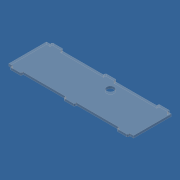
# Autodesk Inventor part: P1704_203
Saved by Autodesk Inventor 2015 (Build 190159000, 159)
## iProperties
Created: 2017-02-08
Part Number: P1704_203
Project: Manette
Material: Plastique PMMA
Description: Paroi avant - Table
Document SubType Name: Modeling
Designer: Alexandre.PICOTTE
Authority: 172x58x3
Density: 1.188 g/cm^3
Appearance: Transparent - Clair
Mass: 33.2535 g
Surface Area: 202.588 cm^2
Volume: 27.9912 cm^3
Material number: ---
Author: Boris.GAUDARD
Autodesk Inventor part; units mm, degrees
ref_plane "Plan YZ" through (0, 0, 0) normal (1, 0, 0) x (0, 1, 0)
ref_plane "Plan XZ" through (0, 0, 0) normal (0, 1, 0) x (-1, 0, 0)
ref_plane "Plan XY" through (0, 0, 0) normal (0, 0, 1) x (1, 0, 0)
sketch "Esquisse12" plane through (0, 0, 0) normal (0, 0, 1) x (1, 0, 0)
  line L0 (-86, -26) -> (-86, 26)
  line L1 (-86, 26) -> (-81, 26)
  line L2 (-81, 26) -> (-81, 29)
  line L3 (-81, 29) -> (-66, 29)
  line L4 (-66, 29) -> (-66, 26)
  line L5 (7.5, 26) -> (7.5, 29)
  line L6 (7.5, 29) -> (-7.5, 29)
  line L7 (-7.5, 29) -> (-7.5, 26)
  line L8 (66, 26) -> (66, 29)
  line L9 (66, 29) -> (81, 29)
  line L10 (81, 29) -> (81, 26)
  line L11 (81, 26) -> (86, 26)
  line L12 (86, 26) -> (86, -26)
  line L13 (86, -26) -> (81, -26)
  line L14 (81, -26) -> (81, -29)
  line L15 (81, -29) -> (66, -29)
  line L16 (66, -29) -> (66, -26)
  line L17 (-7.5, -26) -> (-7.5, -29)
  line L18 (7.5, -29) -> (7.5, -26)
  line L19 (-66, -26) -> (-66, -29)
  line L20 (-81, -29) -> (-81, -26)
  line L21 (-86, -26) -> (-81, -26)
  line L22 (-81, -29) -> (-66, -29)
  line L23 (7.5, -29) -> (-7.5, -29)
  line L24 (-66, 26) -> (-7.5, 26)
  line L25 (7.5, 26) -> (66, 26)
  line L26 (7.5, -26) -> (66, -26)
  line L27 (-7.5, -26) -> (-66, -26)
  line L28 (-120.4, 0) -> (120.4, 0) construction
  line L29 (0, -40.6) -> (0, 40.6) construction
  point P0 (0, 0)
  dimension "d86" = 52
  dimension "d87" = 3
  dimension "d88" = 5
  dimension "d90" = 15
  dimension "d112" = 172
  constraints: 56 end point, 27 point on line, 10 perpendicular, 7 equal length, 3 collinear, 2 parallel, 2 vertical, 1 horizontal, 2 other
  measures "d86" distance of L0.start L0.end
  measures "d87" distance of L1.end L2.end
  measures "d88" distance of L0.end L1.end
  measures "d90" distance of L2.end L3.end
  measures "d112" distance between parallel lines of L12 L0
extrude "Extrusion5" add sketch "Esquisse12" along normal blind 3
sketch "Esquisse13" plane through (0, 0, 3) normal (0, 0, 1) x (1, 0, 0)
  point P0 (0, 0)
  point P1 (-81, 26)
  point P2 (-66, 26)
  point P3 (-81, -26)
  point P4 (-66, -26)
  point P5 (-7.5, -26)
  point P6 (7.5, -26)
  point P7 (66, -26)
  point P8 (81, -26)
  point P9 (81, 26)
  point P10 (66, 26)
  point P11 (-7.5, 26)
  point P12 (7.5, 26)
hole "Perçage6" at (-81, 26, 3) at (-66, 26, 3) at (-81, -26, 3) at (-66, -26, 3) at (-7.5, -26, 3) at (7.5, -26, 3) at (66, -26, 3) at (81, -26, 3) at (81, 26, 3) at (66, 26, 3) at (-7.5, 26, 3) at (7.5, 26, 3) direction (0, 0, -1) diameter 1 end through all
chamfer "Chanfrein3" distance 1 angle 45 12 edges at (-81, 29, 1.5) (-66, 29, 1.5) (-7.5, 29, 1.5) (7.5, 29, 1.5) (66, 29, 1.5) (81, 29, 1.5) (-81, -29, 1.5) (-66, -29, 1.5) (-7.5, -29, 1.5) (7.5, -29, 1.5) (66, -29, 1.5) (81, -29, 1.5)
sketch "Esquisse14" plane through (0, 0, 3) normal (0, 0, 1) x (1, 0, 0)
  circle A0 centre (14.3, 13.8) radius 5
  line L0 (-86, -26) -> (-86, 26) projected
  line L1 (65.5, -26) -> (8, -26) projected
  point P0 (0, 0)
  dimension "d107" = 100.3
  dimension "d108" = 39.8
  dimension "d109" = 10
  constraints: 1 centre point
  measures "d107" distance from line of L0 A0.centre
  measures "d108" distance from line of L1 A0.centre
  measures "d109" diameter of A0
extrude "Extrusion6" cut sketch "Esquisse14" against normal through all
